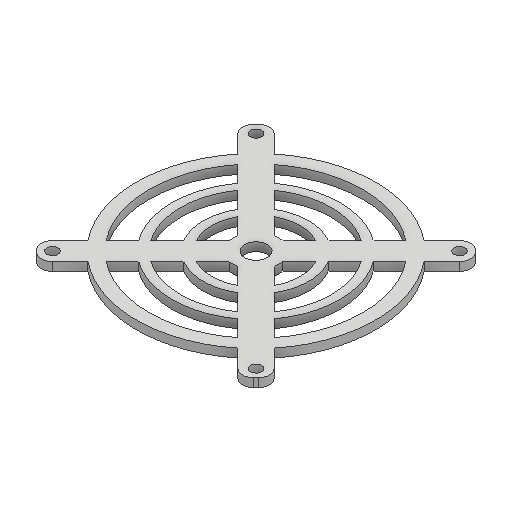
# Autodesk Inventor part: 3DP_PLA_Controller_Case_Fan_Grill
Saved by Autodesk Inventor 2026.1 (Build 301233000, 233)
## iProperties
Created: 2017-05-27
Part Number: 3DP_PLA_Controller_Case_Fan_Grill
Material: Ogólny
Document SubType Name: Modeling
Designer: Andrzej
Density: 1 g/cm^3
Appearance: Domyślna
Mass: 10.0715 g
Surface Area: 104.806 cm^2
Volume: 10.0715 cm^3
Author: Andrzej
Autodesk Inventor part; units mm, degrees
ref_plane "YZ Plane" through (0, 0, 0) normal (1, 0, 0) x (0, 1, 0)
ref_plane "XZ Plane" through (0, 0, 0) normal (0, 1, 0) x (-1, 0, 0)
ref_plane "XY Plane" through (0, 0, 0) normal (0, 0, 1) x (1, 0, 0)
sketch "Szkic1" plane through (0, 0, 0) normal (0, 0, 1) x (1, 0, 0)
  circle A0 centre (41.8843, 27.3116) radius 37.5
  circle A1 centre (41.8843, 27.3116) radius 42
  circle A2 centre (41.8843, 27.3116) radius 29.5
  circle A3 centre (41.8843, 27.3116) radius 26.5
  circle A4 centre (41.8843, 27.3116) radius 18.5
  circle A5 centre (41.8843, 27.3116) radius 15.5
  circle A6 centre (41.8843, 27.3116) radius 8
  line L0 (0.1239, 62.7081) -> (6.4879, 69.072)
  line L1 (83.6448, 62.7081) -> (77.2808, 69.072)
  line L2 (77.2808, -14.4488) -> (83.6448, -8.0848)
  line L3 (0.1239, -8.0848) -> (6.4879, -14.4488)
  line L4 (0.1239, 62.7081) -> (77.2808, -14.4488)
  line L5 (6.4879, 69.072) -> (83.6448, -8.0848)
  line L6 (0.1239, -8.0848) -> (77.2808, 69.072)
  line L7 (6.4879, -14.4488) -> (83.6448, 62.7081)
  point P0 (0, 0)
  point P1 (0, 0)
  point P2 (6.1343, 63.0616)
  point P3 (77.6343, 63.0616)
  point P4 (77.6343, -8.4384)
  point P5 (6.1343, -8.4384)
  dimension "d0" = 75
  dimension "d1" = 35.75
  dimension "d2" = 35.75
  dimension "d3" = 35.75
  dimension "d4" = 35.75
  dimension "d5" = 35.75
  dimension "d6" = 35.75
  dimension "d7" = 35.75
  dimension "d8" = 35.75
  dimension "d9" = 4.5
  dimension "d20" = 8
  dimension "d21" = 3
  dimension "d22" = 8
  dimension "d23" = 3
  dimension "d24" = 16
  dimension "d33" = 4
  dimension "d34" = 4
  dimension "d35" = 4
  dimension "d36" = 4
  constraints: 16 end point, 7 centre point, 1 coincident, 1 perpendicular
  measures "d0" diameter of A0
  measures "d1" horizontal distance of point (6.134, 63.062) A0.centre
  measures "d2" horizontal distance of A0.centre point (6.134, 63.062)
  measures "d3" horizontal distance of A0.centre point (6.134, -8.438)
  measures "d4" horizontal distance of A0.centre point (6.134, -8.438)
  measures "d5" horizontal distance of point (77.634, 63.062) A0.centre
  measures "d6" horizontal distance of A0.centre point (77.634, 63.062)
  measures "d7" horizontal distance of A0.centre point (77.634, -8.438)
  measures "d8" horizontal distance of A0.centre point (77.634, -8.438)
  measures "d9" radial gap between concentric circles of A0 A1
  measures "d20" radial gap between concentric circles of A0 A2
  measures "d21" radial gap between concentric circles of A2 A3
  measures "d22" radial gap between concentric circles of A3 A4
  measures "d23" radial gap between concentric circles of A4 A5
  measures "d24" diameter of A6
  measures "d33" distance from line of L0 point (6.134, 63.062)
  measures "d34" distance from line of L1 point (77.634, 63.062)
  measures "d35" distance from line of L3 point (6.134, -8.438)
  measures "d36" distance from line of L2 point (77.634, -8.438)
extrude "Wyciągnięcie proste1" add sketch "Szkic1" along normal blind 3 contours A0 L7 A1 L5 | L7 A2 L6 A0 | A0 L6 A1 L7 | L5 A1 L4 A0 | A0 L4 A2 L5 | A0 L5 A1 L6 | L7 A3 L6 A2 | A2 L5 A3 L7 | A1 L6 L1 L7 | L4 A1 L7 A0 | A2 L4 A3 L5 | L5 L2 L4 A1 | L5 A2 L4 A0 | A0 L4 A1 L5 | L6 A3 L5 A2 | L7 A4 L6 A3 | L7 A1 L6 A0 | A0 L6 A2 L7 | A2 L7 A3 L4 | A3 L4 A4 L5 | A0 L6 A1 L4 | A1 L4 L0 L5 | L5 A3 L4 A2 | L7 A5 L6 A4 | A4 L5 A5 L7 | L7 L3 L6 A1 | A2 L6 A3 L7 | A4 L4 A5 L5 | L4 A3 L6 A2 | L5 A4 L4 A3 | L6 A5 L5 A4 | L7 A6 L6 A5 | A3 L6 A4 L7 | A4 L7 A5 L4 | A5 L4 A6 L5 | L5 A5 L4 A4 | L7 L5 L6 A6 | A6 L5 L7 | A4 L6 A5 L7 | A6 L4 L7 L5 | L4 A5 L6 A4 | L5 A6 L4 A5 | L6 L5 A6 | L7 L4 L6 L5 | A5 L6 A6 L7 | A6 L7 L4 | L5 L6 L4 A6 | L7 A6 L6 L4 | L4 L6 A6
hole "Otwór1" at (6.1343, -8.4384, 0) at (77.6343, -8.4384, 0) at (77.6343, 63.0616, 0) at (6.1343, 63.0616, 0) direction (0, 0, 1) diameter 4 end through all
fillet "Zaokrąglenie1" radius 4 8 edges at (6.4879, -14.4488, 1.5) (0.1239, -8.0848, 1.5) (77.2808, -14.4488, 1.5) (83.6448, -8.0848, 1.5) (83.6448, 62.7081, 1.5) (77.2808, 69.072, 1.5) (0.1239, 62.7081, 1.5) (6.4879, 69.072, 1.5)
hole "Otwór2" at (41.8843, 27.3116, 0) direction (0, 0, 1) diameter 8 depth 8 tip angle 118
equation "\"d2\" = d1"
equation "\"d3\" = d1"
equation "\"d4\" = d1"
equation "\"d5\" = d1"
equation "\"d6\" = d1"
equation "\"d7\" = d1"
equation "\"d8\" = d1"
equation "\"d17\" = d16"
equation "\"d18\" = d16"
equation "\"d19\" = d16"
equation "\"d16\" = 4.5"
